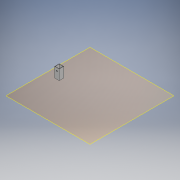
# Autodesk Inventor part: ステア棒
Saved by Autodesk Inventor 2018 (Build 220112000, 112)
## iProperties
Created: 2017-09-20
Part Number: ステア棒
Material: 一般
Document SubType Name: Modeling
Designer: mura5
Density: 1 g/cm^3
Appearance: 既定
Author: mura5
Autodesk Inventor part; units mm, degrees
ref_plane "YZ Plane" through (0, 0, 0) normal (1, 0, 0) x (0, 1, 0)
ref_plane "XZ Plane" through (0, 0, 0) normal (0, 1, 0) x (-1, 0, 0)
ref_plane "XY Plane" through (0, 0, 0) normal (0, 0, 1) x (1, 0, 0)
sketch "スケッチ2" plane through (0, 0, 0) normal (0, 1, 0) x (-1, 0, 0)
  line L0 (43, -215) -> (-441.4, 962.3333)
  line L1 (32, 0) -> (32, -200)
  line L2 (0, 0) -> (0, -200)
  line L3 (32, 0) -> (0, 0)
  line L4 (16, 0) -> (16, -149.3765)
  line L5 (32, -200) -> (0, -200)
  dimension "d0" = 50.6234
  constraints: 12 end point, 1 midpoint, 1 perpendicular, 1 point on line, 1 vertical
  measures "d0" vertical distance of L1.end L4.end
ref_plane "作業平面1" through (-32, 0, -200) normal (0, 0, 1) x (1, 0, 0)
sketch "スケッチ5" plane through (-32, 0, -200) normal (0, 0, 1) x (1, 0, 0)
  line L0 (0, -16) -> (32, -16)
  line L1 (32, -16) -> (32, 16)
  line L2 (32, 16) -> (0, 16)
  line L3 (0, 16) -> (0, -16)
  line L4 (0, -16) -> (32, 16) construction
  line L5 (32, -16) -> (0, 16) construction
  line L6 (29.7, -13.7) -> (2.3, -13.7)
  line L7 (2.3, -13.7) -> (2.3, 13.7)
  line L8 (2.3, 13.7) -> (29.7, 13.7)
  line L9 (29.7, 13.7) -> (29.7, -13.7)
  point P0 (32, 0)
  point P1 (16, 0)
  dimension "d7" = 32
  dimension "d8" = 32
  dimension "d9" = 2.3
  constraints: 20 end point, 4 parallel, 2 midpoint, 2 perpendicular, 1 horizontal, 3 other
  measures "d7" distance of L2.end L1.end
  measures "d8" distance of L1.end L0.end
  measures "d9" distance between parallel lines of L0 L6
extrude "押し出し2" add sketch "スケッチ5" along normal blind 70
sketch "スケッチ6" plane through (-32, -16, -200) normal (0, -1, 0) x (1, 0, 0)
  line L0 (-11, -15) -> (473.4, 1162.3333) projected
  line L1 (16, 200) -> (16, 50.6235) projected
  point P0 (32, 200)
  constraints: 1 coincident
hole "穴1" at (-16, -16, -149.3765) direction (0, 1, 0) diameter 10 end through all
